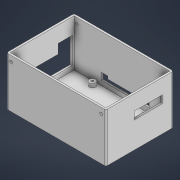
# Autodesk Inventor part: RPIholder
Saved by Autodesk Inventor 2022 (Build 260153000, 153)
## iProperties
Created: 2023-10-20
Part Number: RPIholder
Material: Všeobecné
Document SubType Name: Modeling
Designer: tada
Density: 1 g/cm^3
Appearance: Výchozí
Author: tada
Autodesk Inventor part; units mm, degrees
ref_plane "YZ Plane" through (0, 0, 0) normal (1, 0, 0) x (0, 1, 0)
ref_plane "XZ Plane" through (0, 0, 0) normal (0, 1, 0) x (-1, 0, 0)
ref_plane "XY Plane" through (0, 0, 0) normal (0, 0, 1) x (1, 0, 0)
sketch "Náčrt1" plane through (0, 0, 0) normal (0, 1, 0) x (-1, 0, 0)
  line L0 (0, 0) -> (-106, 0)
  line L1 (-106, 0) -> (-106, -62)
  line L2 (-106, -62) -> (0, -62)
  line L3 (0, -62) -> (0, 0)
  line L4 (-104, -2) -> (-2, -2)
  line L5 (-2, -2) -> (-2, -60)
  line L6 (-2, -60) -> (-104, -60)
  line L7 (-104, -60) -> (-104, -2)
  line L8 (-5.8, 0) -> (-5.8, -18) construction
  circle A0 centre (-5.8, -19.6) radius 1.6
  line L9 (0, -19.6) -> (-4.2, -19.6) construction
  line L10 (-7.4, 0) -> (-7.4, -5.6) construction
  circle A1 centre (-5.8, -5.6) radius 1.6
  line L11 (0, -7.2) -> (-5.8, -7.2) construction
  line L12 (-53, 11.0609) -> (-53, -73.3805) construction
  line L13 (-100.2, 0) -> (-100.2, -18) construction
  circle A2 centre (-100.2, -19.6) radius 1.6
  line L14 (-106, -19.6) -> (-101.8, -19.6) construction
  line L15 (-98.6, 0) -> (-98.6, -5.6) construction
  circle A3 centre (-100.2, -5.6) radius 1.6
  line L16 (-106, -7.2) -> (-100.2, -7.2) construction
  dimension "d0" = 62
  dimension "d1" = 106
  dimension "d2" = 2
  dimension "d8" = 18
  dimension "d9" = 4.2
  dimension "d10" = 3.2
  dimension "d13" = 5.8
  dimension "d14" = 5.6
  dimension "d15" = 3.2
  constraints: 34 end point, 10 symmetric about line, 8 point on circle, 4 centre point, 4 parallel, 4 point on line, 4 vertical, 3 horizontal, 2 line through centre, 2 perpendicular, 2 tangent, 5 other
  measures "d0" distance of L0.end L1.end
  measures "d1" distance of L1.end L2.end
  measures "d2" distance between parallel lines of L0 L4
  measures "d8" distance of L8.start L8.end
  measures "d9" distance of L9.start L9.end
  measures "d10" diameter of A0
  measures "d13" distance of L11.start L11.end
  measures "d14" distance of L10.start L10.end
  measures "d15" diameter of A1
extrude "Vysunutí1" add sketch "Náčrt1" along normal blind 2 contours L4 L5 L6 L7 | A0 | A1 | A2 | A3
extrude "Vysunutí2" add sketch "Náčrt1" along normal blind 52 contours L3 L2 L1 L0
extrude "Vysunutí3" cut sketch "Náčrt1" along normal blind 2 contours A0 | A1 | A2 | A3
sketch "Náčrt2" plane through (0, 2, 0) normal (0, 1, 0) x (1, 0, 0)
  circle A0 centre (84, 55.5) radius 1.3
  line L0 (2, 60) -> (104, 60) projected
  circle A1 centre (26, 55.5) radius 1.3
  line L1 (2, 2) -> (2, 60) projected
  circle A2 centre (26, 6.5) radius 1.3
  circle A3 centre (84, 6.5) radius 1.3
  line L2 (104, 2) -> (2, 2) projected
  circle A4 centre (26, 6.5) radius 3.3
  circle A5 centre (26, 55.5) radius 3.3
  circle A6 centre (84, 55.5) radius 3.3
  circle A7 centre (84, 6.5) radius 3.3
  point P0 (0, 0)
  dimension "d19" = 4.5
  dimension "d20" = 2.6
  dimension "d21" = 2.6
  dimension "d22" = 58
  dimension "d23" = 24
  dimension "d24" = 4.5
  dimension "d25" = 2.6
  dimension "d26" = 24
  dimension "d27" = 2.6
  dimension "d28" = 58
  dimension "d29" = 4.5
  dimension "d30" = 4.5
  dimension "d31" = 49
  dimension "d32" = 2
  dimension "d33" = 2
  dimension "d34" = 2
  dimension "d35" = 2
  constraints: 8 centre point
  measures "d19" distance from line of L0 A0.centre
  measures "d20" diameter of A0
  measures "d21" diameter of A1
  measures "d22" distance of A0.centre A1.centre
  measures "d23" distance from line of L1 A1.centre
  measures "d24" distance from line of A1.centre L0
  measures "d25" diameter of A2
  measures "d26" distance from line of L1 A2.centre
  measures "d27" diameter of A3
  measures "d28" distance of A2.centre A3.centre
  measures "d29" distance from line of L2 A2.centre
  measures "d30" distance from line of L2 A3.centre
  measures "d31" distance of A3.centre A0.centre
  measures "d32" radial gap between concentric circles of A4 A2
  measures "d33" radial gap between concentric circles of A5 A1
  measures "d34" radial gap between concentric circles of A6 A0
  measures "d35" radial gap between concentric circles of A7 A3
extrude "Vysunutí4" add sketch "Náčrt2" along normal blind 4
extrude "Vysunutí5" cut sketch "Náčrt2" against normal blind 2 contours A0 | A1 | A2 | A3
sketch "Náčrt3" plane through (0, 0, -62) normal (-1, 0, 0) x (0, 0, 1)
  line L0 (4, 7) -> (58, 7)
  line L1 (58, 7) -> (58, 25)
  line L2 (58, 25) -> (4, 25)
  line L3 (4, 25) -> (4, 7)
  line L4 (9.8, 6) -> (3.2, 6) projected
  line L5 (2, 2) -> (2, 52) projected
  line L6 (60, 2) -> (60, 52) projected
  point P0 (62, 0)
  dimension "d40" = 1
  dimension "d41" = 54
  dimension "d42" = 18
  dimension "d43" = 2
  dimension "d44" = 2
  constraints: 8 end point, 2 parallel, 1 horizontal, 1 perpendicular
  measures "d40" distance between parallel lines of L0 L4
  measures "d41" distance between parallel lines of L1 L3
  measures "d42" distance between parallel lines of L2 L0
  measures "d43" distance between parallel lines of L5 L3
  measures "d44" distance between parallel lines of L6 L1
extrude "Vysunutí6" cut sketch "Náčrt3" against normal blind 2
sketch "Náčrt4" plane through (106, 0, -62) normal (0, 0, -1) x (-1, 0, 0)
  line L0 (24, 7) -> (75, 7)
  line L1 (75, 7) -> (75, 11.5)
  line L2 (75, 11.5) -> (24, 11.5)
  line L3 (24, 11.5) -> (24, 7)
  line L4 (104, 2) -> (104, 52) projected
  line L5 (75, 11.5) -> (68, 11.5)
  line L6 (68, 11.5) -> (68, 14.5)
  line L7 (68, 14.5) -> (75, 14.5)
  line L8 (75, 14.5) -> (75, 11.5)
  line L9 (2, 2) -> (104, 2) projected
  point P0 (106, 0)
  point P1 (68, 11.5)
  dimension "d47" = 4.5
  dimension "d48" = 29
  dimension "d49" = 51
  dimension "d50" = 5
  dimension "d51" = 7.5
  dimension "d52" = 7
  constraints: 16 end point, 4 parallel, 2 horizontal, 2 perpendicular
  measures "d47" distance between parallel lines of L2 L0
  measures "d48" distance between parallel lines of L1 L4
  measures "d49" distance between parallel lines of L3 L1
  measures "d50" distance between parallel lines of L0 L9
  measures "d51" distance between parallel lines of L0 L7
  measures "d52" distance between parallel lines of L6 L8
extrude "Vysunutí7" cut sketch "Náčrt4" against normal blind 2
sketch "Náčrt5" plane through (0, 0, 0) normal (0, -1, 0) x (1, 0, 0)
  line L0 (106, 0) -> (106, -62) projected
  line L1 (106, -2) -> (0, -2)
  line L2 (0, -2) -> (0, 10)
  line L3 (0, 10) -> (106, 10)
  line L4 (106, 10) -> (106, -2)
  line L5 (2, -2) -> (104, -2) projected
  line L6 (106, 10) -> (0, 10)
  line L7 (0, 10) -> (0, 8)
  line L8 (0, 8) -> (106, 8)
  line L9 (106, 8) -> (106, 10)
  line L10 (104, -60) -> (104, -2) projected
  line L11 (104, -2) -> (106, -2)
  line L12 (106, -2) -> (106, 10)
  line L13 (106, 10) -> (104, 10)
  line L14 (104, 10) -> (104, -2)
  line L15 (2, -2) -> (2, -60) projected
  line L16 (2, -2) -> (0, -2)
  line L17 (0, -2) -> (0, 10)
  line L18 (0, 10) -> (2, 10)
  line L19 (2, 10) -> (2, -2)
  point P0 (0, 0)
  point P1 (2, 8)
  point P2 (104, 8)
  dimension "d55" = 12
  dimension "d56" = 106
  dimension "d57" = 2
  constraints: 32 end point, 8 parallel, 4 horizontal, 4 perpendicular, 2 point on line, 1 collinear
  measures "d55" distance between parallel lines of L3 L1
  measures "d56" distance between parallel lines of L4 L2
  measures "d57" distance between parallel lines of L3 L8
extrude "Vysunutí8" cut sketch "Náčrt5" against normal blind 52 contours L1 L19 L8 L14
extrude "Vysunutí9" add sketch "Náčrt5" against normal blind 2 contours L1 L19 L8 L14
extrude "Vysunutí10" add sketch "Náčrt5" against normal blind 52 contours L0 L1 L14 L8 L4 | L8 L14 L3 L4 | L8 L19 L3 L14 | L1 L2 L8 L19 | L8 L2 L3 L19
sketch "Náčrt6" plane through (0, 0, -62) normal (-1, 0, 0) x (0, 0, 1)
  line L0 (4, 25) -> (58, 25) projected
  line L1 (4, 25) -> (19, 25)
  line L2 (19, 25) -> (19, 35)
  line L3 (19, 35) -> (4, 35)
  line L4 (4, 35) -> (4, 25)
  point P0 (62, 0)
  dimension "d64" = 15
  dimension "d65" = 10
  constraints: 8 end point, 2 parallel, 1 horizontal, 1 perpendicular
  measures "d64" distance between parallel lines of L4 L2
  measures "d65" distance between parallel lines of L3 L0
extrude "Vysunutí11" cut sketch "Náčrt6" against normal blind 4
fillet "Zaoblení1" radius 2 4 edges at (106, 26, -62) (0, 26, -62) (0, 26, 10) (106, 26, 10)
sketch "Náčrt7" plane through (2, 0, 10) normal (0, 0, 1) x (1, 0, 0)
  circle A0 centre (3, 46) radius 1.55
  line L0 (0, 52) -> (102, 52) projected
  line L1 (0, 0) -> (0, 52) projected
  circle A1 centre (99, 46) radius 1.55
  line L2 (102, 52) -> (102, 0) projected
  point P0 (-2, 0)
  dimension "d69" = 3.1
  dimension "d70" = 6
  dimension "d71" = 3
  dimension "d72" = 3.1
  dimension "d73" = 3
  dimension "d74" = 6
  constraints: 2 centre point
  measures "d69" diameter of A0
  measures "d70" distance from line of L0 A0.centre
  measures "d71" distance from line of L1 A0.centre
  measures "d72" diameter of A1
  measures "d73" distance from line of L2 A1.centre
  measures "d74" distance from line of L0 A1.centre
extrude "Vysunutí12" cut sketch "Náčrt7" against normal blind 400
sketch "Náčrt8" plane through (106, 0, 8) normal (1, 0, 0) x (0, 0, -1)
  line L0 (28, 36) -> (58, 36)
  line L1 (58, 36) -> (58, 28)
  line L2 (58, 28) -> (28, 28)
  line L3 (28, 28) -> (28, 36)
  line L4 (70, 0) -> (70, 52) projected
  line L5 (0, 0) -> (68, 0) projected
  point P0 (8, 0)
  dimension "d77" = 12
  dimension "d78" = 30
  dimension "d79" = 8
  dimension "d80" = 28
  constraints: 8 end point, 2 parallel, 1 horizontal, 1 perpendicular
  measures "d77" distance between parallel lines of L1 L4
  measures "d78" distance between parallel lines of L3 L1
  measures "d79" distance between parallel lines of L0 L2
  measures "d80" distance between parallel lines of L5 L2
extrude "Vysunutí13" cut sketch "Náčrt8" against normal blind 52
equation "\"d21\" = d20"
equation "\"d24\" = d19"
equation "\"d25\" = d20"
equation "\"d26\" = d23"
equation "\"d27\" = d20"
equation "\"d28\" = d22"
equation "\"d29\" = d19"
equation "\"d30\" = d19"
equation "\"d33\" = d32"
equation "\"d34\" = d32"
equation "\"d35\" = d32"
